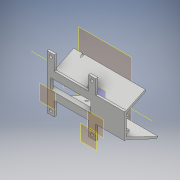
# Autodesk Inventor part: new_cuiller
Saved by Autodesk Inventor 2017 (Build 210142000, 142)
## iProperties
Part Number: new_cuiller
Material: Générique
Document SubType Name: Modeling
Designer: Thomas
Density: 1 g/cm^3
Appearance: Par défaut
Author: Thomas
Autodesk Inventor part; units mm, degrees
ref_plane "YZ Plane" through (0, 0, 0) normal (1, 0, 0) x (0, 1, 0)
ref_plane "XZ Plane" through (0, 0, 0) normal (0, 1, 0) x (-1, 0, 0)
ref_plane "XY Plane" through (0, 0, 0) normal (0, 0, 1) x (1, 0, 0)
ref_plane "Plan de construction16" through (10, -26.1714, -17.6889) normal (0, -1, 0) x (1, 0, 0)
sketch "Esquisse9" plane through (10, -26.1714, -17.6889) normal (0, -1, 0) x (1, 0, 0)
  line L0 (0, 35.3779) -> (8, 35.3779) projected
  line L1 (68, 1.8848) -> (68, 33.493) projected
  line L2 (0, 35.3779) -> (68, 35.3779)
  line L3 (68, 35.3779) -> (68, 32.0585)
  line L4 (0, 32.0585) -> (0, 35.3779)
  line L5 (0, 0) -> (8, 0) projected
  line L6 (0, 37.6889) -> (0, -2.3111) projected
  line L7 (68, 0) -> (0, 0)
  line L8 (0, 0) -> (0, 3.3237)
  line L9 (68, 3.3237) -> (68, 0)
  line L10 (68, 35.3779) -> (0, 35.3779)
  line L11 (0, 35.3779) -> (0, 0)
  line L12 (0, 0) -> (68, 0)
  line L13 (68, 0) -> (68, 35.3779)
  point P0 (-10, 17.6889)
  point P1 (67.75, 35.3779)
  point P2 (67.75, 0)
  constraints: 20 end point, 4 parallel, 3 horizontal, 3 perpendicular, 2 point on line
extrude "Extrusion11" add sketch "Esquisse9" against normal blind 3
ref_plane "Plan de construction18" through (78, -26.1714, -17.6889) normal (0, -1, 0) x (1, 0, 0)
sketch "Esquisse13" plane through (78, -26.1714, -17.6889) normal (0, -1, 0) x (1, 0, 0)
  line L0 (-65, 35.3779) -> (-60, 35.3779) projected
  line L1 (0, 35.3779) -> (-10, 35.3779)
  line L2 (-10, 35.3779) -> (-10, 55.3779)
  line L3 (-10, 55.3779) -> (0, 55.3779)
  line L4 (0, 55.3779) -> (0, 35.3779)
  line L5 (0, 35.3779) -> (0, 0) construction
  line L6 (0, 17.6889) -> (-68.1792, 17.6889) construction
  line L7 (-68.1792, 35.3779) -> (-58.1792, 35.3779)
  line L8 (-58.1792, 35.3779) -> (-58.1792, 55.3779)
  line L9 (-58.1792, 55.3779) -> (-68.1792, 55.3779)
  line L10 (-68.1792, 55.3779) -> (-68.1792, 35.3779)
  line L11 (-65, 0) -> (0, 0)
  line L12 (0, 0) -> (-10, 0)
  line L13 (-10, 0) -> (-10, -20)
  line L14 (-10, -20) -> (0, -20)
  line L15 (0, -20) -> (0, 0)
  line L16 (-68.1792, 0) -> (-58.1792, 0)
  line L17 (-58.1792, 0) -> (-58.1792, -20)
  line L18 (-58.1792, -20) -> (-68.1792, -20)
  line L19 (-68.1792, -20) -> (-68.1792, 0)
  line L20 (-5, 34.0863) -> (-5, 43.2092) construction
  circle A0 centre (-5, 50.3779) radius 2.25
  circle A1 centre (-63.1792, 50.3779) radius 2.25
  circle A2 centre (-63.1792, -15) radius 2.25
  line L21 (-5, -1.4113) -> (-5, -11.1612) projected
  circle A3 centre (-5, -15) radius 2.25
  point P0 (-78, 17.6889)
  point P1 (0, 1.8848)
  point P2 (0, 33.493)
  point P3 (-0.25, 35.3779)
  dimension "d45" = 10
  dimension "d46" = 20
  dimension "d47" = 10
  dimension "d48" = 20
  dimension "d49" = 4.5
  dimension "d50" = 4.5
  dimension "d51" = 4.5
  dimension "d52" = 4.5
  dimension "d57" = 0
  dimension "d58" = 5
  dimension "d59" = 5
  dimension "d60" = 5
  dimension "d61" = 5
  constraints: 36 end point, 9 symmetric about line, 4 centre point, 4 parallel, 3 horizontal, 2 perpendicular, 2 point on line, 1 midpoint
  measures "d45" distance of L2.end L3.end
  measures "d46" distance of L1.end L2.end
  measures "d47" distance of L9.end L8.end
  measures "d48" distance of L8.end L7.end
  measures "d49" diameter of A0
  measures "d50" diameter of A1
  measures "d51" diameter of A2
  measures "d52" diameter of A3
  measures "d57" distance between parallel lines of L0 L7
  measures "d58" distance from line of L9 A1.centre
  measures "d59" distance from line of A0.centre L3
  measures "d60" distance from line of L14 A3.centre
  measures "d61" distance from line of L18 A2.centre
extrude "Extrusion12" add sketch "Esquisse13" against normal blind 3
ref_plane "Plan de construction19" through (18, 0, 0) normal (1, 0, 0) x (0, 0, -1)
sketch "Esquisse14" plane through (18, 0, 0) normal (1, 0, 0) x (0, 0, -1)
  line L0 (-19.134, -23.1714) -> (-15.8041, -23.1714)
  line L1 (-19.134, -23.1714) -> (-15.8041, -23.1714) projected
  line L2 (-15.8041, -23.1714) -> (-36.599, 20) projected
  line L3 (-38.4838, 17) -> (-19.134, -23.1714) projected
  line L4 (-19.134, -23.1714) -> (-15.8041, -23.1714) projected
  line L5 (-19.134, -23.1714) -> (-15.8041, -23.1714) projected
  line L6 (-36.599, 20) -> (-38.4838, 17) projected
  line L7 (-15.8041, -23.1714) -> (-36.599, 20) projected
  line L8 (-36.599, 20) -> (-38.4838, 17) projected
  line L9 (-38.4838, 17) -> (-19.134, -23.1714) projected
  line L10 (-15.8041, -23.1714) -> (-36.599, 20) projected
  line L11 (-36.599, 20) -> (-38.4838, 17) projected
  line L12 (-38.4838, 17) -> (-19.134, -23.1714) projected
  line L13 (17.6889, -23.1714) -> (-17.6889, -23.1714) projected
  line L14 (-14.4365, -23.1714) -> (-35.9022, 21.1089)
  line L15 (-35.9022, 21.1089) -> (-36.599, 20)
  line L16 (0, 22.9524) -> (0, -23.1714) construction
  line L17 (15.8041, -23.1714) -> (36.599, 20)
  line L18 (-17.6889, -23.1714) -> (17.6889, -23.1714)
  line L19 (14.4365, -23.1714) -> (35.9022, 21.1089)
  line L20 (35.9022, 21.1089) -> (36.599, 20)
  line L21 (14.4365, -23.1714) -> (15.8041, -23.1714)
  line L22 (35.9022, 21.1089) -> (36.599, 20)
  line L23 (15.8041, -23.1714) -> (36.599, 20)
  line L24 (35.9022, 21.1089) -> (14.4365, -23.1714)
  line L25 (-36.599, 20) -> (-37.5414, 18.5)
  line L26 (-17.6889, -23.1714) -> (-17.6889, -26.1714) projected
  line L27 (-37.5414, 18.5) -> (-17.6889, -23.1714)
  line L28 (-17.6889, -23.1714) -> (-14.4365, -23.1714)
  line L29 (35.9022, 21.1089) -> (37.5414, 18.5)
  line L30 (37.5414, 18.5) -> (17.4582, -23.1714)
  line L31 (14.4365, -23.1714) -> (17.4582, -23.1714)
  point P0 (0, 0)
  constraints: 36 end point, 7 symmetric about line, 6 collinear, 3 point on line, 2 midpoint, 1 perpendicular
ref_plane "Plan de construction10" through (78, -23.1714, 15.8041) normal (0, 1, 0) x (1, 0, 0)
sketch "Esquisse15" plane through (78, -23.1714, 15.8041) normal (0, 1, 0) x (1, 0, 0)
  line L0 (0, 53.493) -> (0, -21.8848) projected
  line L1 (-68, 5.6727) -> (0, 5.6727)
  line L2 (0, 5.6727) -> (0, 8.3531)
  line L3 (0, 8.3531) -> (-68, 8.3531)
  line L4 (-68, 8.3531) -> (-68, 5.6727)
  line L5 (-68, 33.493) -> (-68, -1.8848) projected
  line L6 (-68, -1.8848) -> (-68, 33.493) construction
  line L7 (-68, 15.8041) -> (0, 15.8041) construction
  line L8 (0, 53.493) -> (0, -21.8848)
  line L9 (-68, 25.9355) -> (0, 25.9355)
  line L10 (0, 25.9355) -> (0, 23.255)
  line L11 (0, 23.255) -> (-68, 23.255)
  line L12 (-68, 23.255) -> (-68, 25.9355)
  line L13 (-68, -1.8848) -> (-68, 33.493)
  line L14 (-68, 33.493) -> (-68, -1.8848) construction
  point P0 (-78, 15.8041)
  constraints: 24 end point, 8 symmetric about line, 2 midpoint, 2 parallel, 2 point on line, 1 collinear, 1 horizontal, 1 perpendicular
extrude "Extrusion14" add sketch "Esquisse15" along normal blind 4 contours L0 L11 L5 L9 | L0 L1 L4 L3
ref_plane "Plan de construction11" through (68, -26.1714, -37.6889) normal (0, -1, 0) x (1, 0, 0)
sketch "Esquisse16" plane through (68, -26.1714, -37.6889) normal (0, -1, 0) x (1, 0, 0)
  line L0 (-58, 45.1399) -> (10, 45.1399) projected
  line L1 (-58, 30.238) -> (10, 30.238) projected
  line L2 (3.117, 45.1399) -> (-52.8886, 45.1399)
  line L3 (-52.8886, 45.1399) -> (-52.8886, 30.238)
  line L4 (-52.8886, 30.238) -> (3.117, 30.238)
  line L5 (3.117, 30.238) -> (3.117, 45.1399)
  point P0 (-68, 37.6889)
  constraints: 8 end point, 2 parallel, 2 point on line, 1 horizontal, 1 perpendicular
extrude "Extrusion15" cut sketch "Esquisse16" against normal blind 4
extrude "Extrusion16" add sketch "Esquisse14" along normal up to surface (60 mm away) contours L19 L20 L17 L13 | L27 L6 L2 L0 | L2 L15 L14 L13 | L17 L29 L30 L13
ref_plane "Plan de construction20" through (18, 21.1089, -35.9022) normal (0, -1, 0) x (1, 0, 0)
sketch "Esquisse17" plane through (18, 21.1089, -35.9022) normal (0, -1, 0) x (1, 0, 0)
  circle A0 centre (18.615, 35.9022) radius 22.5 construction
  circle A1 centre (45.1277, 16.765) radius 1.25
  line L0 (50, 53.5912) -> (50, 73.5912) projected
  circle A2 centre (13.6149, 6.5446) radius 1.25
  line L1 (60, 43.3532) -> (60, 28.4513) projected
  line L2 (-11.4468, 35.9022) -> (31.8074, 35.9022) construction
  circle A3 centre (45.1277, 55.0395) radius 1.25
  line L3 (13.6149, 53.5912) -> (50, -1.7867)
  circle A4 centre (13.6149, 65.2599) radius 1.25
  point P0 (-18, 35.9022)
  dimension "d68" = 45
  dimension "d69" = 2.5
  dimension "d70" = 2.5
  dimension "d71" = 41.385
  constraints: 5 centre point, 4 end point, 1 horizontal, 1 symmetric about line
  measures "d68" diameter of A0
  measures "d69" diameter of A1
  measures "d70" diameter of A2
  measures "d71" distance from line of L1 A0.centre
extrude "Extrusion17" cut sketch "Esquisse17" along normal up to surface (44.2803 mm away)
sketch "Esquisse18" plane through (18, 21.1089, -35.9022) normal (0, -1, 0) x (1, 0, 0)
  line L0 (-5.0895, 79.4289) -> (61.3071, 79.4289)
  line L1 (61.3071, 79.4289) -> (61.3071, 14.8125)
  line L2 (61.3071, 14.8125) -> (-5.0895, 14.8125)
  line L3 (-5.0895, 14.8125) -> (-5.0895, 79.4289)
  point P0 (-18, 35.9022)
  constraints: 8 end point, 2 parallel, 1 horizontal, 1 perpendicular
extrude "Extrusion18" cut sketch "Esquisse18" along normal blind 18
sketch "Esquisse19" plane through (78, -26.1714, 37.6889) normal (1, 0, 0) x (0, 0, -1)
  line L0 (10.5125, 29.2803) -> (7.4799, 29.2803) projected
  line L1 (20, 3) -> (7.4799, 29.2803) projected
  line L2 (0, 3) -> (20, 3) projected
  line L3 (0, 0) -> (0, 3) projected
  line L4 (75.3779, 0) -> (0, 0) projected
  line L5 (75.3779, 0) -> (75.3779, 3) projected
  line L6 (55.1472, 3) -> (75.3779, 3) projected
  line L7 (75.2303, 44.6714) -> (55.1472, 3) projected
  line L8 (73.5912, 47.2803) -> (75.2303, 44.6714) projected
  line L9 (52.1254, 3) -> (73.5912, 47.2803) projected
  line L10 (47.8203, 3) -> (52.1254, 3) projected
  line L11 (47.8203, 3) -> (47.8203, 7) projected
  line L12 (45.1399, 7) -> (47.8203, 7) projected
  line L13 (45.1399, 3) -> (45.1399, 7) projected
  line L14 (30.238, 3) -> (45.1399, 3) projected
  line L15 (30.238, 3) -> (30.238, 7) projected
  line L16 (27.5576, 7) -> (30.238, 7) projected
  line L17 (27.5576, 3) -> (27.5576, 7) projected
  line L18 (23.2524, 3) -> (27.5576, 3) projected
  line L19 (10.5125, 29.2803) -> (23.2524, 3) projected
  line L20 (0, 3) -> (20, 3) projected
  line L21 (20, 3) -> (20, 0) projected
  line L22 (20, 0) -> (55.3779, 0) projected
  line L23 (55.1472, 3) -> (75.2303, 44.6714) projected
  line L24 (47.8203, 0) -> (50.6711, 0)
  line L25 (20, 3) -> (20, 0)
  line L26 (20, 0) -> (55.1472, 0)
  line L27 (55.1472, 3) -> (55.1472, 0)
  line L28 (55.1472, 3) -> (75.2303, 44.6714)
  point P0 (37.6889, 26.1714)
  constraints: 10 end point, 3 collinear, 3 point on line, 1 perpendicular
extrude "Extrusion19" add sketch "Esquisse19" along normal blind 40 contours L19 L18 L17 L16 L15 L14 L13 L12 L11 L10 L9 L8 L7 L27 L4 L21 L1 L0
